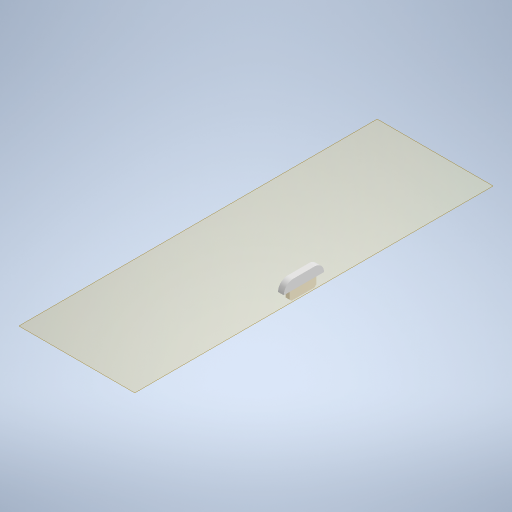
# Autodesk Inventor part: zatic
Saved by Autodesk Inventor 2024 (Build 280153000, 153)
## iProperties
Created: 2023-09-16
Part Number: zatic
Material: Generic
Document SubType Name: Modeling
Designer: jebes windows
Density: 1 g/cm^3
Appearance: Default
Author: jebes windows
Autodesk Inventor part; units mm, degrees
ref_plane "YZ Plane" through (0, 0, 0) normal (1, 0, 0) x (0, 1, 0)
ref_plane "XZ Plane" through (0, 0, 0) normal (0, 1, 0) x (-1, 0, 0)
ref_plane "XY Plane" through (0, 0, 0) normal (0, 0, 1) x (1, 0, 0)
ref_plane "Work Plane1" through (0, 0, 0) normal (0, 0, 1) x (1, 0, 0)
sketch "Sketch1" plane through (0, 0, 0) normal (0, 0, 1) x (1, 0, 0)
  line L0 (94.5, 7.5) -> (97.5, 7.5) projected
  line L1 (97.5, 7.5) -> (97.5, -7.5) projected
  line L2 (97.5, -7.5) -> (94.5, -7.5) projected
  line L3 (94.5, -7.5) -> (94.5, 7.5) projected
  line L4 (45, -80) -> (45, 63.0557) projected
  line L5 (90, -80) -> (45, -80) projected
  line L6 (90, -80) -> (90, -85) projected
  arc A0 (90, -85) -> (100, -75) centre (90, -75) ccw projected
  line L7 (100, -75) -> (100, 75) projected
  arc A1 (100, 75) -> (90, 85) centre (90, 75) ccw projected
  line L8 (90, 85) -> (90, 80) projected
  line L9 (61.9443, 80) -> (90, 80) projected
  arc A2 (45, 63.0557) -> (61.9443, 80) centre (53, 72) ccw projected
  line L10 (97.5, -7.5) -> (97.5, -10.5)
  line L11 (97.5, -10.5) -> (94.5, -10.5)
  line L12 (94.5, -10.5) -> (94.5, -7.5)
  line L13 (94.5, 7.5) -> (94.5, 10.5)
  line L14 (94.5, 10.5) -> (97.5, 10.5)
  line L15 (97.5, 10.5) -> (97.5, 7.5)
  point P0 (0, 0)
  dimension "d0" = 3
  dimension "d1" = 3
  constraints: 12 end point, 4 perpendicular, 2 vertical
  measures "d0" distance of L1.end L10.end
  measures "d1" distance of L0.start L13.end
extrude "Extrusion1" add sketch "Sketch1" along normal blind 5 contours L13 L14 L15 L0 | L0 L1 L2 L3 | L2 L10 L11 L12
sketch "Sketch2" plane through (0, 0, 0) normal (0, 0, -1) x (-1, 0, 0)
  line L0 (-97.5, 7.5) -> (-94.5, 7.5) projected
  line L1 (-94.5, 7.5) -> (-94.5, -7.5) projected
  line L2 (-94.5, -7.5) -> (-97.5, -7.5) projected
  line L3 (-97.5, -7.5) -> (-97.5, 7.5) projected
  circle A0 centre (-53, 72) radius 10 projected
  circle A1 centre (-20, 0) radius 10 projected
  arc A2 (100, 75) -> (90, 85) centre (90, 75) ccw projected
  line L4 (-90, 85) -> (90, 85) projected
  arc A3 (-90, 85) -> (-100, 75) centre (-90, 75) ccw projected
  line L5 (-100, -75) -> (-100, 75) projected
  arc A4 (-100, -75) -> (-90, -85) centre (-90, -75) ccw projected
  line L6 (90, -85) -> (-90, -85) projected
  arc A5 (90, -85) -> (100, -75) centre (90, -75) ccw projected
  line L7 (100, 75) -> (100, -75) projected
  line L8 (-95, -7) -> (-95, 7)
  line L9 (-95, 7) -> (-97, 7)
  line L10 (-97, 7) -> (-97, -7)
  line L11 (-97, -7) -> (-95, -7)
  point P0 (0, 0)
  dimension "d4" = 0.5
  constraints: 8 end point, 3 other
  measures "d4" distance between parallel lines of L1 L8
ref_plane "Work Plane2" through (-147.9274, -141.3852, -5) normal (0, 0, -1) x (0, 1, 0)
extrude "Extrusion2" add sketch "Sketch2" along normal up to surface (5 mm away) contours L11 L10 L9 L8
fillet "Fillet1" radius 5 2 edges at (96, 10.5, 5) (96, -10.5, 5)
chamfer "Chamfer1" distance 1 angle 45 2 edges at (96, 7, -5) (96, -7, -5)
body "Solid1"
